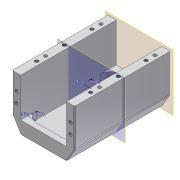
# Autodesk Inventor part: J002876
Saved by Autodesk Inventor 2012 SP2 (Build 160219200, 219)
## iProperties
Created: 2014-07-29
Material: ALUMINUM, 6061-T651
Vendor: HHMI: JFRC - ID&F
Document SubType Name: Modeling
Designer: arnoldj
Density: 1 g/cm^3
Part Number: J002876
Description: MPS Sling
Project: P-194005
RuleStatus: InUse
AfterDocSave0: file://Part Number Cleaner
LAB/DEPT: SVOBODA (LAB)
REQUESTING SCIENTIST: PERON, SIMON
SURFACE ROUGHNESS: 63 Ra
DESIGN DEPARTMENT: HHMI: JFRC - ID&F
SPECIAL FINISH: ANODIZE PER MIL-A-8625F, TYPE II, CLASS 2 (BLACK)
ALTERED ITEM PART NUMBER: N/A
ALTERED ITEM VENDOR: N/A
ALTERED ITEM DESCRIPTION: N/A
Revision Number: -
Autodesk Inventor part; units mm, degrees
ref_plane "YZ Plane" through (0, 0, 0) normal (1, 0, 0) x (0, 1, 0)
ref_plane "Work Plane3" through (0, 0, -43.815) normal (0, 0, 1) x (1, 0, 0)
sketch "Sketch1" plane through (0, 0, 0) normal (0, 0, 1) x (1, 0, 0)
  line L0 (0, 76.2) -> (0, -12.7) projected
  line L1 (-40.005, 0) -> (40.005, 0) projected
  line L2 (-28.575, 0) -> (28.575, 0)
  line L3 (28.575, 0) -> (28.575, 47.625)
  line L4 (-28.575, 47.625) -> (-28.575, 0)
  line L5 (-20.955, 47.625) -> (-20.955, 5.08)
  line L6 (-20.955, 5.08) -> (20.955, 5.08)
  line L7 (20.955, 5.08) -> (20.955, 47.625)
  line L8 (28.575, 47.625) -> (20.955, 47.625)
  line L9 (-20.955, 47.625) -> (-28.575, 47.625)
  point P0 (0, 0)
  point P1 (0, 63.5)
  dimension "d0" = 57.15
  dimension "d1" = 47.625
  dimension "d4" = 7.62
  dimension "d5" = 7.62
  dimension "d7" = 5.08
  dimension "d43" = 41.91
  constraints: 16 end point, 4 parallel, 4 perpendicular, 1 horizontal, 1 horizontal alignment, 1 point on line, 1 vertical alignment, 1 other
  measures "d0" distance of L3.end L4.start
  measures "d1" distance of L4.start L2.start
  measures "d4" distance of L5.start L4.start
  measures "d5" distance of L3.end L7.end
  measures "d7" distance between parallel lines of L6 L1
  measures "d43" distance of L5.end L6.end
extrude "Extrusion1" add sketch "Sketch1" along normal mid plane 87.63
ref_plane "Work Plane1" through (0, 47.625, 0) normal (0, 1, 0) x (-1, 0, 0)
sketch "Sketch2" plane through (0, 47.625, 0) normal (0, 1, 0) x (-1, 0, 0)
  line L0 (0, -61.341) -> (0, 61.341) projected
  line L1 (-40.005, 0) -> (40.005, 0) projected
  line L2 (-24.765, 17.145) -> (24.765, 17.145)
  line L3 (24.765, 17.145) -> (24.765, -33.655)
  line L4 (24.765, -33.655) -> (-24.765, -33.655)
  line L5 (-24.765, -33.655) -> (-24.765, 17.145)
  line L6 (20.955, 43.815) -> (-20.955, 43.815) projected
  line L7 (-20.955, -43.815) -> (20.955, -43.815) projected
  line L8 (-28.575, -43.815) -> (-28.575, 43.815) projected
  line L9 (28.575, -43.815) -> (28.575, 43.815) projected
  point P0 (0, 0)
  point P1 (0, 17.145)
  dimension "d9" = 49.53
  dimension "d10" = 50.8
  dimension "d57" = 33.655
  constraints: 8 end point, 2 parallel, 1 horizontal, 1 midpoint, 1 perpendicular, 1 vertical alignment
  measures "d9" distance of L2.start L2.end
  measures "d10" distance of L4.end L2.start
  measures "d57" distance between parallel lines of L1 L4
hole "Hole1 Locating pins" at (-24.765, 47.625, 17.145) at (-24.765, 47.625, -33.655) at (24.765, 47.625, -33.655) at (24.765, 47.625, 17.145) direction (0, -1, 0) diameter 3.1623 depth 10.795 tip angle 118 counterbore diameter 3.2004 counterbore depth 1.905
sketch "Sketch3" plane through (0, 47.625, 0) normal (0, 1, 0) x (-1, 0, 0)
  line L0 (0, -61.341) -> (0, 61.341) projected
  line L1 (-40.005, 0) -> (40.005, 0) projected
  line L2 (-24.765, 25.4) -> (24.765, 25.4)
  line L3 (24.765, 25.4) -> (24.765, -25.4)
  line L4 (24.765, -25.4) -> (-24.765, -25.4)
  line L5 (-24.765, -25.4) -> (-24.765, 25.4)
  point P0 (0, 0)
  point P1 (-24.765, 0)
  point P2 (0, 25.4)
  point P3 (-24.765, 0)
  point P4 (24.765, 0)
  dimension "d18" = 49.53
  dimension "d19" = 50.8
  constraints: 8 end point, 3 midpoint, 2 parallel, 1 coincident, 1 horizontal, 1 horizontal alignment, 1 perpendicular, 1 vertical alignment
  measures "d18" distance of L2.start L2.end
  measures "d19" distance of L4.end L2.start
hole "Hole2 M4 Tapped" at (24.765, 47.625, -25.4) at (24.765, 47.625, 25.4) at (-24.765, 47.625, 25.4) at (-24.765, 47.625, -25.4) at (24.765, 47.625, 0) at (-24.765, 47.625, 0) direction (0, -1, 0) diameter 3.2512 depth 9.525 tip angle 118
sketch "Sketch4" plane through (-20.955, 5.08, 43.815) normal (0, 1, 0) x (1, 0, 0)
  line L0 (0, 0) -> (41.91, 0) projected
  line L1 (41.91, 87.63) -> (0, 87.63) projected
  line L2 (41.91, 87.63) -> (41.91, 0) projected
  line L3 (0, 87.63) -> (41.91, 87.63)
  line L4 (41.91, 87.63) -> (41.91, 82.55)
  line L5 (41.91, 82.55) -> (0, 82.55)
  line L6 (0, 82.55) -> (0, 87.63)
  line L7 (0, 0) -> (41.91, 0)
  line L8 (41.91, 0) -> (41.91, 5.08)
  line L9 (41.91, 5.08) -> (0, 5.08)
  line L10 (0, 5.08) -> (0, 0)
  point P0 (20.955, 43.815)
  dimension "d27" = 5.08
  dimension "d28" = 5.08
  constraints: 16 end point, 4 parallel, 2 horizontal, 2 perpendicular, 2 point on line
  measures "d27" distance of L5.end L1.end
  measures "d28" distance of L7.end L8.end
extrude "Extrusion2" add sketch "Sketch4" along normal blind 6.858
fillet "Fillet1" radius 9.525 4 edges at (-20.955, 8.509, -38.735) (20.955, 8.509, -38.735) (20.955, 8.509, 38.735) (-20.955, 8.509, 38.735)
sketch "Sketch5" plane through (0, 0, 0) normal (0, 1, 0) x (-1, 0, 0)
  circle A0 centre (0, 0) radius 1.27
  line L0 (-28.575, -43.815) -> (-28.575, 43.815) projected
  line L1 (28.575, -43.815) -> (28.575, 43.815) projected
  dimension "d32" = 2.54
  dimension "d44" = 28.575
  dimension "d45" = 28.575
  constraints: 1 centre point, 1 coincident
  measures "d32" diameter of A0
  measures "d44" distance from line of point (0, 0) L0
  measures "d45" distance from line of L1 point (0, 0)
hole "Hole3" at (0, 0, 0) direction (0, 1, 0) diameter 4.9276 end through all
fillet "Fillet2" [suppressed]
chamfer "Chamfer2" [suppressed]
sketch "Sketch6" plane through (0, 0, 0) normal (0, 1, 0) x (-1, 0, 0)
  circle A0 centre (24.765, -33.655) radius 1.5685 projected
  circle A1 centre (24.765, -25.4) radius 1.6256 projected
  circle A2 centre (24.765, 25.4) radius 1.6256 projected
  circle A3 centre (24.765, 17.145) radius 1.5685 projected
  point P0 (0, 0)
  dimension "d55" = 8.255
  dimension "d56" = 8.255
  measures "d55" distance of A0.centre A1.centre
  measures "d56" distance of A2.centre A3.centre
sketch "Sketch7" plane through (0, 0, 0) normal (0, 0, 1) x (1, 0, 0)
  line L0 (0, 9.144) -> (0, -1.524) projected
  line L1 (-33.4467, 0) -> (15.9461, 0) projected
  point P0 (0, 0)
  point P1 (-8.89, 7.62)
  point P2 (8.89, 7.62)
  dimension "d58" = 17.78
  dimension "d59" = 8.89
  dimension "d60" = 7.62
  constraints: 1 horizontal alignment
  measures "d58" distance of point (8.89, 7.62) point (-8.89, 7.62)
  measures "d59" distance from line of L0 point (-8.89, 7.62)
  measures "d60" distance from line of L1 point (-8.89, 7.62)
hole "Hole4" [suppressed]
mirror "Mirror1" [suppressed]
sketch "Sketch8" plane through (0, 0, -43.815) normal (0, 0, 1) x (1, 0, 0)
  line L0 (24.765, 32.9184) -> (-24.765, 32.9184) construction
  line L1 (-24.765, 32.9184) -> (-24.765, 23.3934) construction
  line L2 (-24.765, 23.3934) -> (24.765, 23.3934) construction
  line L3 (24.765, 23.3934) -> (24.765, 32.9184) construction
  line L4 (28.575, 0) -> (28.575, 47.625) construction
  line L5 (-28.575, 47.625) -> (-28.575, 0) construction
  line L6 (28.575, 47.625) -> (20.955, 47.625) construction
  point P0 (0, 0)
  point P1 (28.575, 12.7)
  point P2 (-28.575, 12.7)
  dimension "d69" = 3.81
  dimension "d70" = 3.81
  dimension "d71" = 9.525
  dimension "d72" = 14.7066
  constraints: 8 end point, 4 coincident, 2 parallel, 1 horizontal, 1 perpendicular
  measures "d69" distance between parallel lines of L3 L4
  measures "d70" distance between parallel lines of L1 L5
  measures "d71" distance of L2.end L0.start
  measures "d72" distance between parallel lines of L0 L6
hole "Hole5" at (24.765, 32.9184, -43.815) at (24.765, 23.3934, -43.815) at (-24.765, 23.3934, -43.815) at (-24.765, 32.9184, -43.815) direction (0, 0, 1) diameter 3.2512 depth 10.795 tip angle 118
mirror "Mirror2" about plane through (0, 0, 0) normal (0, 0, 1) of "Hole5"
chamfer "Chamfer3" distance 7.62 distance2 12.7 1 edges at (-28.575, 0, 0) measured on face at (-28.075, 0, 0)
chamfer "Chamfer4" distance 7.62 distance2 12.7 1 edges at (28.575, 0, 0) measured on face at (28.075, 0, 0)
fillet "Fillet3" radius 3.175 4 edges at (28.575, 12.7, 0) (20.955, 0, 0) (-20.955, 0, 0) (-28.575, 12.7, 0)
chamfer "Chamfer5" distance 0.635 angle 45 18 edges at (0, 0, 43.815) (-20.7217, 0.4121, 43.815) (-25.0012, 6.7437, 43.815) (-28.4598, 12.7319, 43.815) (-28.575, 30.6022, 43.815) (20.7217, 0.4121, 43.815) (25.0012, 6.7437, 43.815) (28.4598, 12.7319, 43.815) (28.575, 30.6022, 43.815) (0, 0, -43.815) (20.7217, 0.4121, -43.815) (25.0012, 6.7437, -43.815) (28.4598, 12.7319, -43.815) (28.575, 30.6022, -43.815) (-20.7217, 0.4121, -43.815) (-25.0012, 6.7437, -43.815) (-28.4598, 12.7319, -43.815) (-28.575, 30.6022, -43.815)
ref_plane "Work Plane2" through (0, 0, 0) normal (0, 0, 1) x (1, 0, 0)
ref_plane "Work Plane4" through (0, 0, 0) normal (0, 0, 1) x (1, 0, 0)
equation "\"d59\" = 0.5 * d58"
body "Solid1"
